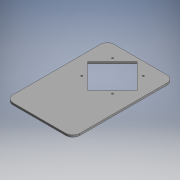
# Autodesk Inventor part: Part7
Saved by Autodesk Inventor 2019.2 (Build 232265000, 265)
## iProperties
Part Number: Part7
Material: Generic
Document SubType Name: Modeling
Designer: richard.girt
Mass: 31.0087 g
Surface Area: 240.873 cm^2
Volume: 31.0087 cm^3
Density: 1 g/cm^3
Appearance: Default
Author: richard.girt
Autodesk Inventor part; units mm, degrees
ref_plane "YZ Plane" through (0, 0, 0) normal (1, 0, 0) x (0, 1, 0)
ref_plane "XZ Plane" through (0, 0, 0) normal (0, 1, 0) x (-1, 0, 0)
ref_plane "XY Plane" through (0, 0, 0) normal (0, 0, 1) x (1, 0, 0)
sketch "Sketch1" plane through (0, 0, 0) normal (0, 1, 0) x (-1, 0, 0)
  line L0 (-47.5, 72) -> (47.5, 72)
  line L1 (47.5, 72) -> (47.5, -72)
  line L2 (47.5, -72) -> (-47.5, -72)
  line L3 (-47.5, -72) -> (-47.5, 72)
  line L4 (-47.5, 72) -> (47.5, -72) construction
  line L5 (47.5, 72) -> (-47.5, -72) construction
  line L6 (0, 3.3553) -> (35.3553, -32)
  line L7 (35.3553, -32) -> (0, -67.3553)
  line L8 (0, -67.3553) -> (-35.3553, -32)
  line L9 (-35.3553, -32) -> (0, 3.3553)
  line L10 (0, 3.3553) -> (0, -67.3553) construction
  line L11 (35.3553, -32) -> (-35.3553, -32) construction
  point P0 (0, 0)
  point P1 (0, -32)
  point P2 (0, -32)
  point P3 (0, 0)
  dimension "d0" = 95
  dimension "d1" = 144
  dimension "d2" = 50
  dimension "d3" = 40
  constraints: 24 end point, 6 midpoint, 4 parallel, 3 perpendicular, 1 horizontal, 1 vertical, 1 vertical alignment
  measures "d0" distance of L0.start L0.end
  measures "d1" distance of L0.end L1.end
  measures "d2" distance of L7.end L8.end
  measures "d3" distance from line of point (0, -32) L2
extrude "Extrusion1" add sketch "Sketch1" along normal blind 2.8
sketch "Sketch2" plane through (0, 2.8, 0) normal (0, 1, 0) x (1, 0, 0)
  line L0 (-35.3553, 32) -> (0, 67.3553) construction
  line L1 (0, 67.3553) -> (35.3553, 32) construction
  line L2 (35.3553, 32) -> (0, -3.3553) construction
  line L3 (0, -3.3553) -> (-35.3553, 32) construction
  line L4 (0, 75.8406) -> (-43.8406, 32)
  line L5 (-43.8406, 32) -> (0, -11.8406)
  line L6 (0, -11.8406) -> (43.8406, 32)
  line L7 (43.8406, 32) -> (0, 75.8406)
  point P0 (0, 0)
  point P1 (-21.9203, 53.9203)
  point P2 (21.9203, 53.9203)
  point P3 (21.9203, 10.0797)
  point P4 (-21.9203, 10.0797)
  dimension "d6" = 6
  constraints: 8 end point, 4 midpoint, 3 other
  measures "d6" distance between parallel lines of L1 L7
hole "Hole1" at (-21.9203, 2.8, -53.9203) at (21.9203, 2.8, -53.9203) at (21.9203, 2.8, -10.0797) at (-21.9203, 2.8, -10.0797) direction (0, -1, 0) diameter 2.5 end through all
fillet "Fillet1" radius 10 4 edges at (-47.5, 1.4, 72) (47.5, 1.4, 72) (47.5, 1.4, -72) (-47.5, 1.4, -72)
body "Solid1"
